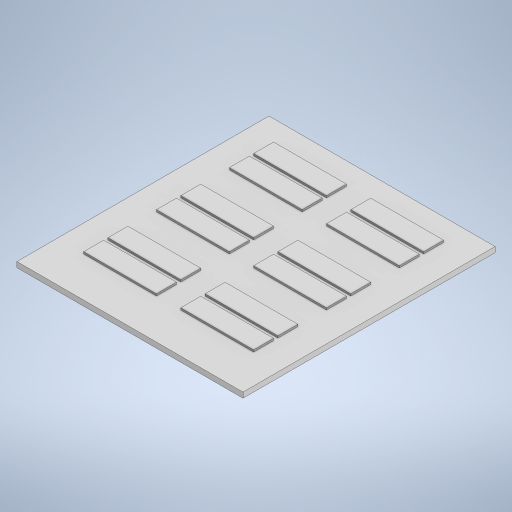
# Autodesk Inventor part: AcrilicoY
Saved by Autodesk Inventor 2024 (Build 280153000, 153)
## iProperties
Created: 2023-06-26
Part Number: AcrilicoY
Material: Genérico
Document SubType Name: Modeling
Designer: Personal
Density: 2.32417 g/cm^3
Appearance: Valor por defecto
Mass: 395.3 g
Surface Area: 807.757 cm^2
Volume: 170.083 cm^3
Author: Personal
Autodesk Inventor part; units mm, degrees
ref_plane "YZ Plane" through (0, 0, 0) normal (1, 0, 0) x (0, 1, 0)
ref_plane "XZ Plane" through (0, 0, 0) normal (0, 1, 0) x (-1, 0, 0)
ref_plane "Plano de trabajo1" through (0, 0, 0) normal (0, 0, 1) x (1, 0, 0)
sketch "Boceto1" plane through (0, 0, 0) normal (0, 0, 1) x (1, 0, 0)
  line L0 (97.5, 97.5) -> (-97.5, 97.5) construction
  line L1 (93.1, -97.5) -> (93.1, 97.5) construction
  line L2 (-93.1, -97.5) -> (-93.1, 97.5) construction
  line L3 (93.1, 93.1) -> (-93.1, 93.1)
  line L4 (-93.1, 93.1) -> (-93.1, 97.5)
  line L5 (-93.1, 97.5) -> (93.1, 97.5)
  line L6 (93.1, 97.5) -> (93.1, 93.1)
  point P0 (0, 0)
  dimension "d0" = 4.4
  constraints: 8 end point, 2 parallel, 1 horizontal, 1 perpendicular, 1 point on line
  measures "d0" distance between parallel lines of L0 L3
extrude "Extrusión1" add sketch "Boceto1" along normal blind 207.6
sketch "Boceto2" plane through (-93.1, 97.5, 0) normal (0, 1, 0) x (1, 0, 0)
  line L0 (22.0667, -18.252) -> (82.0667, -18.252)
  line L1 (82.0667, -18.252) -> (82.0667, -34.7233)
  line L2 (82.0667, -34.7233) -> (22.0667, -34.7233)
  line L3 (22.0667, -34.7233) -> (22.0667, -18.252)
  line L4 (102.0667, -18.252) -> (162.0667, -18.252)
  line L5 (162.0667, -18.252) -> (162.0667, -34.7233)
  line L6 (162.0667, -34.7233) -> (102.0667, -34.7233)
  line L7 (102.0667, -34.7233) -> (102.0667, -18.252)
  line L8 (22.0667, -38.252) -> (82.0667, -38.252)
  line L9 (82.0667, -38.252) -> (82.0667, -54.7233)
  line L10 (82.0667, -54.7233) -> (22.0667, -54.7233)
  line L11 (22.0667, -54.7233) -> (22.0667, -38.252)
  line L12 (102.0667, -38.252) -> (162.0667, -38.252)
  line L13 (162.0667, -38.252) -> (162.0667, -54.7233)
  line L14 (162.0667, -54.7233) -> (102.0667, -54.7233)
  line L15 (102.0667, -54.7233) -> (102.0667, -38.252)
  line L16 (0, 0) -> (0, -207.6) projected
  line L17 (82.0667, -114.7233) -> (22.0667, -114.7233)
  line L18 (22.0667, -78.252) -> (82.0667, -78.252)
  line L19 (82.0667, -78.252) -> (82.0667, -94.7233)
  line L20 (22.0667, -94.7233) -> (22.0667, -78.252)
  line L21 (22.0667, -98.252) -> (82.0667, -98.252)
  line L22 (82.0667, -98.252) -> (82.0667, -114.7233)
  line L23 (22.0667, -114.7233) -> (22.0667, -98.252)
  line L24 (102.0667, -94.7233) -> (102.0667, -78.252)
  line L25 (102.0667, -114.7233) -> (102.0667, -98.252)
  line L26 (102.0667, -78.252) -> (162.0667, -78.252)
  line L27 (162.0667, -78.252) -> (162.0667, -94.7233)
  line L28 (162.0667, -98.252) -> (162.0667, -114.7233)
  line L29 (162.0667, -114.7233) -> (102.0667, -114.7233)
  line L30 (102.0667, -98.252) -> (162.0667, -98.252)
  line L31 (162.0667, -94.7233) -> (102.0667, -94.7233)
  line L32 (82.0667, -94.7233) -> (22.0667, -94.7233)
  line L33 (82.0667, -174.7233) -> (22.0667, -174.7233)
  line L34 (22.0667, -138.252) -> (82.0667, -138.252)
  line L35 (82.0667, -138.252) -> (82.0667, -154.7233)
  line L36 (22.0667, -154.7233) -> (22.0667, -138.252)
  line L37 (22.0667, -158.252) -> (82.0667, -158.252)
  line L38 (82.0667, -158.252) -> (82.0667, -174.7233)
  line L39 (22.0667, -174.7233) -> (22.0667, -158.252)
  line L40 (102.0667, -154.7233) -> (102.0667, -138.252)
  line L41 (102.0667, -174.7233) -> (102.0667, -158.252)
  line L42 (102.0667, -138.252) -> (162.0667, -138.252)
  line L43 (162.0667, -138.252) -> (162.0667, -154.7233)
  line L44 (162.0667, -158.252) -> (162.0667, -174.7233)
  line L45 (162.0667, -174.7233) -> (102.0667, -174.7233)
  line L46 (102.0667, -158.252) -> (162.0667, -158.252)
  line L47 (162.0667, -154.7233) -> (102.0667, -154.7233)
  line L48 (82.0667, -154.7233) -> (22.0667, -154.7233)
  point P0 (93.1, 0)
  dimension "d5" = 80
  dimension "d8" = 20
  dimension "d11" = 22.0667
  dimension "d12" = 60
  dimension "d15" = 60
  constraints: 96 end point, 2 collinear, 2 horizontal, 2 parallel, 2 vertical, 1 perpendicular, 86 other
  measures "d5" distance of L0.start L4.start
  measures "d8" distance of L0.start L8.start
  measures "d11" distance between parallel lines of L16 L3
  measures "d12" distance of L0.start L0.end
  measures "d15" distance of L0.start L18.start
extrude "Extrusión2" add sketch "Boceto2" along normal blind 1.6
